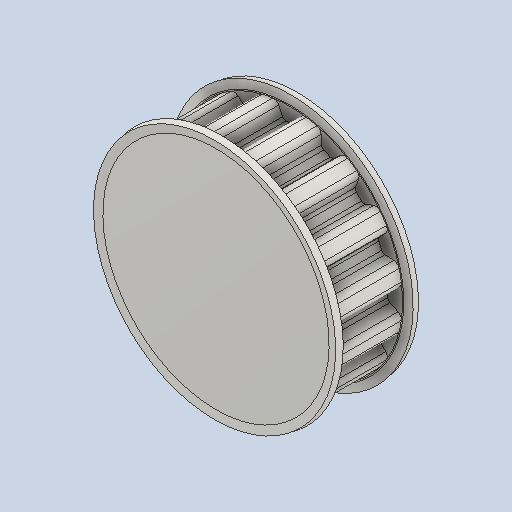
# Autodesk Inventor part: 歯付きプーリ3
Saved by Autodesk Inventor 2025.2 (Build 292293000, 293)
## iProperties
CustomPartVersion: 1
Created: 2025-04-09
Part Number: 歯付きプーリ3
Material: Steel
Document SubType Name: Modeling
Designer: haruy
Density: 1 g/cm^3
Appearance: Steel
Author: haruy
Autodesk Inventor part; units mm, degrees
ref_plane "YZ Plane" through (0, 0, 0) normal (1, 0, 0) x (0, 1, 0)
ref_plane "XZ Plane" through (0, 0, 0) normal (0, 1, 0) x (-1, 0, 0)
ref_plane "XY Plane" through (0, 0, 0) normal (0, 0, 1) x (1, 0, 0)
sketch "プーリ スケッチ" plane through (0, 0, 0) normal (0, 0, 1) x (1, 0, 0)
  circle A0 centre (0, 0) radius 12.9361 construction
  circle A1 centre (0, 0) radius 12.6821
  circle A2 centre (0, 0) radius 11.0311
  line L0 (-1.3944, 12.6052) -> (-0.6604, 11.0311)
  line L1 (-0.6604, 11.0311) -> (0.6604, 11.0311)
  line L2 (0.6604, 11.0311) -> (1.3944, 12.6052)
  line L3 (0, 0) -> (0, 12.6821) construction
  point P0 (0, 11.0311)
  dimension "d0" = 25.8722
  dimension "d1" = 0.254
  dimension "d2" = 1.651
  dimension "d3" = 50
  dimension "d4" = 1.3208
  constraints: 8 end point, 3 coincident, 3 point on circle, 2 centre point, 1 horizontal, 1 midpoint, 1 point on line, 1 vertical, 1 vertical alignment, 3 other
  measures "d0" diameter of A0
  measures "d1" radial gap between concentric circles of A0 A1
  measures "d3" angle of L2 L0
  measures "d4" distance of L0.end L1.end
extrude "基本ボディ" add sketch "プーリ スケッチ" along normal mid plane 7.5 contours A2 | A1 L0 L1 L2 | L2 L1 L0 A1
extrude "歯" cut sketch "プーリ スケッチ" along normal through all both and the other way through all contours L2 L1 L0 A1 picked at (0, 12.1261)
fillet "Fillet" radius 0.4064 2 edges at (0.6604, 11.0311, 0) (-0.6604, 11.0311, 0)
fillet "Fillet" radius 0.635 4 edges at (-1.3944, 12.6052, 1.875) (-1.3944, 12.6052, -1.875) (1.3944, 12.6052, 1.875) (1.3944, 12.6052, -1.875)
pattern_circular "Teeth" count 16 over 360 about axis through (0, 0, -10) along (0, 0, 1) of "歯", "Fillet"
pulley flange "左フランジ" diameter 25.3642 height 1.016 thickness 0.7366 bend angle 10 centre (0, 0, -3.75) toward (0, 0, -1)
pulley flange "右フランジ" diameter 25.3642 height 1.016 thickness 0.7366 bend angle 10 centre (0, 0, 3.75) toward (0, 0, 1)
equation "\"d1\" = da_a"
equation "\"d2\" = da_hg"
equation "\"d3\" = 2 * da_fi"
equation "\"d4\" = da_bw"
equation "\"d5\" = da_bf"
equation "\"d7\" = da_bf"
equation "\"d9\" = da_rb"
equation "\"d10\" = da_rt"
equation "\"da_pb\" = 5.08"
equation "\"da_fi\" = 25deg"
equation "\"da_hg\" = 1.651"
equation "\"da_bw\" = 1.3208"
equation "\"da_rb\" = 0.4064"
equation "\"da_rt\" = 0.635"
equation "\"da_a\" = 0.254"
equation "\"da_bf\" = 7.5"
equation "\"da_wf\" = 0.7366"
equation "\"da_hf\" = 1.016"
body "Solid1"
